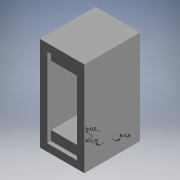
# Autodesk Inventor part: Upper_leg
Saved by Autodesk Inventor 2017 (Build 210142000, 142)
## iProperties
Part Number: Upper_leg
Material: Generic
Document SubType Name: Modeling
Designer: alex-
Appearance: Generic
Author: alex-
Autodesk Inventor part; units mm, degrees
ref_plane "YZ Plane" through (0, 0, 0) normal (1, 0, 0) x (0, 1, 0)
ref_plane "XZ Plane" through (0, 0, 0) normal (0, 1, 0) x (-1, 0, 0)
ref_plane "XY Plane" through (0, 0, 0) normal (0, 0, 1) x (1, 0, 0)
sketch "Sketch1" plane through (0, 0, 0) normal (0, 1, 0) x (-1, 0, 0)
  line L0 (15, 18.75) -> (-15, 18.75)
  line L1 (-15, 18.75) -> (-15, -18.75)
  line L2 (-15, -18.75) -> (15, -18.75)
  line L3 (15, -18.75) -> (15, 18.75)
  point P0 (0, 0)
  point P1 (15, 0)
  point P2 (0, 18.75)
  dimension "d0" = 37.5
  dimension "d1" = 30
  constraints: 8 end point, 2 midpoint, 2 parallel, 1 horizontal, 1 horizontal alignment, 1 perpendicular, 1 vertical alignment
  measures "d0" distance of L2.end L0.start
  measures "d1" distance of L0.end L0.start
extrude "Extrusion1" add sketch "Sketch1" along normal blind 63.5
sketch "Sketch2" plane through (-15, 0, 18.75) normal (0, 0, 1) x (1, 0, 0)
  line L0 (5, 52) -> (25, 52)
  line L1 (25, 52) -> (25, 11.5)
  line L2 (25, 11.5) -> (5, 11.5)
  line L3 (5, 11.5) -> (5, 52)
  line L4 (0, 0) -> (30, 0) projected
  point P0 (15, 0)
  point P1 (15, 11.5)
  point P2 (15, 0)
  dimension "d4" = 40.5
  dimension "d5" = 20
  dimension "d6" = 11.5
  constraints: 8 end point, 2 midpoint, 2 parallel, 1 horizontal, 1 perpendicular, 1 vertical alignment
  measures "d4" distance of L2.end L0.start
  measures "d5" distance of L0.start L0.end
  measures "d6" distance between parallel lines of L4 L2
extrude "Extrusion2" cut sketch "Sketch2" against normal blind 30
sketch "Sketch3" plane through (-15, 0, 18.75) normal (0, 0, 1) x (1, 0, 0)
  line L0 (5, 11.5) -> (25, 11.5)
  line L1 (25, 11.5) -> (25, 5)
  line L2 (25, 5) -> (5, 5)
  line L3 (5, 5) -> (5, 11.5)
  line L4 (5, 58.5) -> (25, 58.5)
  line L5 (25, 58.5) -> (25, 52)
  line L6 (25, 52) -> (5, 52)
  line L7 (5, 52) -> (5, 58.5)
  point P0 (15, 0)
  dimension "d9" = 6.5
  constraints: 16 end point, 4 parallel, 3 coincident, 2 horizontal, 2 perpendicular, 2 point on line, 1 collinear
  measures "d9" distance of L2.end L0.start
extrude "Extrusion3" cut sketch "Sketch3" against normal blind 2.5
sketch "Sketch4" plane through (0, 0, 0) normal (0, -1, 0) x (1, 0, 0)
  line L0 (-3.75, -5.75) -> (3.75, -5.75)
  line L1 (3.75, -5.75) -> (3.75, -10.75)
  line L2 (3.75, -10.75) -> (-3.75, -10.75)
  line L3 (-3.75, -10.75) -> (-3.75, -5.75)
  line L4 (15, -18.75) -> (-15, -18.75) projected
  point P0 (0, 0)
  point P1 (0, -5.75)
  dimension "d12" = 5
  dimension "d13" = 7.5
  dimension "d14" = 8
  constraints: 8 end point, 2 parallel, 1 horizontal, 1 midpoint, 1 perpendicular, 1 vertical alignment
  measures "d12" distance of L2.end L0.start
  measures "d13" distance of L0.start L0.end
  measures "d14" distance between parallel lines of L4 L2
equation "\"d0\" = b_mat_thickness + s_height - s_land_dist_top + s_land_thickness"
equation "\"d1\" = s_depth + 2 * b_mat_thickness"
equation "\"d2\" = 2 * b_mat_thickness + s_width + 2 * s_land"
equation "\"d4\" = s_width"
equation "\"d5\" = s_depth"
equation "\"d6\" = s_land + b_mat_thickness"
equation "\"d7\" = s_height - s_land_dist_top"
equation "\"d9\" = s_land"
equation "\"d10\" = s_land_thickness"
equation "\"d12\" = s_cable_height"
equation "\"d13\" = s_cable_width"
equation "\"d14\" = s_cable_dist_bottom + b_mat_thickness"
equation "\"b_mat_thickness\" = 5"
equation "\"s_height\" = 38"
equation "\"s_land_dist_top\" = 8"
equation "\"s_land_thickness\" = 2.5"
equation "\"s_depth\" = 20"
equation "\"s_width\" = 40.5"
equation "\"s_land\" = 6.5"
equation "\"s_cable_height\" = 5"
equation "\"s_cable_width\" = 7.5"
equation "\"s_cable_dist_bottom\" = 3"
body "Solid1"
